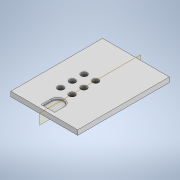
# Autodesk Inventor part: Part2
Saved by Autodesk Inventor 2022.6 (Build 266554010, 554A)
## iProperties
Created: 2025-05-13
Part Number: Part2
Material: Generic
Document SubType Name: Modeling
Designer: khinm
Density: 1 g/cm^3
Appearance: Default
Author: khinm
Autodesk Inventor part; units mm, degrees
ref_plane "XZ Plane" through (0, 0, 0) normal (0, 1, 0) x (-1, 0, 0)
ref_plane "XY Plane" through (0, 0, 0) normal (0, 0, 1) x (1, 0, 0)
sketch "Sketch1" plane through (0, 0, 0) normal (0, 0, 1) x (1, 0, 0)
  line L0 (-37.75, 2.75) -> (37.75, 2.75)
  line L1 (37.75, 2.75) -> (37.75, -2.75)
  line L2 (37.75, -2.75) -> (-37.75, -2.75)
  line L3 (-37.75, -2.75) -> (-37.75, 2.75)
  point P0 (0, 0)
  point P1 (0, 2.75)
  point P2 (-37.75, 0)
  dimension "d0" = 5.5
  dimension "d1" = 75.5
  constraints: 8 end point, 2 midpoint, 2 parallel, 1 horizontal, 1 horizontal alignment, 1 perpendicular, 1 vertical alignment
  measures "d0" distance of L0.end L1.end
  measures "d1" distance of L0.start L0.end
extrude "Extrusion1" add sketch "Sketch1" along normal mid plane 103.5
ref_plane "Work Plane1" through (0, 0, 0) normal (1, 0, 0) x (0, 1, 0)
sketch "Sketch6" plane through (0, 0, 0) normal (1, 0, 0) x (0, 1, 0)
  line L0 (-2.75, 51.75) -> (-2.75, -51.75) projected
  line L1 (-2.75, 49.5) -> (-4.75, 48.3453)
  line L2 (-4.75, 48.3453) -> (-4.75, 47.6547)
  line L3 (-4.75, 47.6547) -> (-2.75, 46.5)
  line L4 (-2.75, 46.5) -> (-2.75, 49.5)
  point P0 (0, 0)
  point P1 (-2.75, 48)
  point P2 (-4.75, 48)
  dimension "d17" = 2.25
  dimension "d18" = 3
  dimension "d19" = 2
  dimension "d20" = 60
  constraints: 8 end point, 2 midpoint, 2 parallel, 1 horizontal alignment, 1 point on line
  measures "d17" distance of L1.start L0.start
  measures "d18" distance of L3.end L1.start
  measures "d19" distance of point (-2.75, 48) point (-4.75, 48)
  measures "d20" angle of L0 L1
extrude "Extrusion4" add sketch "Sketch6" along normal mid plane 59.9
sketch "Sketch7" plane through (-37.75, 2.75, 51.75) normal (0, 1, 0) x (1, 0, 0)
  line L0 (75.5, 0) -> (0, 0) projected
  line L1 (44.3814, 15) -> (44.3814, 5)
  line L2 (44.3814, 5) -> (31.1186, 5)
  line L3 (31.1186, 5) -> (31.1186, 15)
  arc A0 (44.3814, 15) -> (31.1186, 15) centre (37.75, 15) ccw
  point P0 (37.75, 51.75)
  point P1 (37.75, 5)
  point P2 (37.75, 0)
  point P3 (37.75, 0)
  dimension "d23" = 5
  dimension "d25" = 10
  dimension "d26" = 6.6314
  constraints: 6 end point, 3 midpoint, 2 parallel, 2 point on circle, 2 vertical alignment, 1 centre point, 1 horizontal alignment
  measures "d23" distance between parallel lines of L2 L0
  measures "d25" distance of L1.end L1.start
  measures "d26" radius of A0
extrude "Extrusion5" cut sketch "Sketch7" against normal blind 2
chamfer "Chamfer2" distance 1 angle 45 4 edges at (0, 2.75, 30.1186) (6.6314, 2.75, 41.75) (-6.6314, 2.75, 41.75) (0, 2.75, 46.75)
sketch "Sketch8" plane through (-37.75, 2.75, 51.75) normal (0, 1, 0) x (1, 0, 0)
  line L0 (0, 103.5) -> (75.5, 103.5) projected
  line L1 (3, 100.5) -> (72.5, 100.5)
  line L2 (72.5, 100.5) -> (72.5, 6)
  line L3 (72.5, 6) -> (3, 6)
  line L4 (3, 6) -> (3, 100.5)
  line L5 (0, 103.5) -> (0, 0) projected
  line L6 (75.5, 0) -> (0, 0) projected
  line L7 (9.25, 96.25) -> (66.25, 96.25)
  line L8 (66.25, 96.25) -> (66.25, 10.25)
  line L9 (66.25, 10.25) -> (9.25, 10.25)
  line L10 (9.25, 10.25) -> (9.25, 96.25)
  line L11 (18.25, 71.25) -> (44.25, 71.25)
  line L12 (44.25, 71.25) -> (44.25, 18.25)
  line L13 (44.25, 18.25) -> (18.25, 18.25)
  line L14 (18.25, 18.25) -> (18.25, 71.25)
  line L15 (18.25, 44.75) -> (44.25, 44.75)
  line L16 (18.25, 58) -> (44.25, 58)
  line L17 (18.25, 31.5) -> (44.25, 31.5)
  circle A0 centre (24.75, 58) radius 3
  circle A1 centre (24.75, 44.75) radius 3
  circle A2 centre (24.75, 31.5) radius 3
  circle A3 centre (37.75, 58) radius 3
  circle A4 centre (37.75, 44.75) radius 3
  circle A5 centre (37.75, 31.5) radius 3
  point P0 (37.75, 51.75)
  point P1 (37.75, 100.5)
  point P2 (37.75, 103.5)
  point P3 (37.75, 96.25)
  point P4 (3, 53.25)
  point P5 (9.25, 53.25)
  point P6 (31.25, 31.5)
  dimension "d32" = 3
  dimension "d33" = 3
  dimension "d34" = 6
  dimension "d35" = 57
  dimension "d36" = 86
  dimension "d37" = 8
  dimension "d38" = 53
  dimension "d39" = 26
  dimension "d40" = 22
  dimension "d44" = 6.5
  dimension "d45" = 6.5
  dimension "d46" = 6.5
  dimension "d47" = 6.5
  dimension "d48" = 6.5
  dimension "d49" = 6.5
  dimension "d50" = 6
  dimension "d51" = 6
  dimension "d52" = 6
  dimension "d53" = 6
  dimension "d54" = 6
  dimension "d55" = 6
  dimension "d56" = 13.25
  dimension "d57" = 26.5
  dimension "d58" = 13.25
  constraints: 30 end point, 10 point on line, 8 midpoint, 6 centre point, 6 coincident, 6 parallel, 5 perpendicular, 3 horizontal, 2 vertical alignment, 1 horizontal alignment
  measures "d32" distance between parallel lines of L0 L1
  measures "d33" distance between parallel lines of L5 L4
  measures "d34" distance between parallel lines of L3 L6
  measures "d35" distance of L7.start L7.end
  measures "d36" distance of L7.end L8.end
  measures "d37" distance between parallel lines of L13 L9
  measures "d38" distance of L11.end L12.end
  measures "d39" distance of L12.end L13.end
  measures "d40" distance between parallel lines of L8 L12
  measures "d44" distance of L16.start point (24.75, 58)
  measures "d45" distance of L16.end point (37.75, 58)
  measures "d46" distance of L15.start point (24.75, 44.75)
  measures "d47" distance of L15.end point (37.75, 44.75)
  measures "d48" distance of L17.start point (24.75, 31.5)
  measures "d49" distance of L17.end point (37.75, 31.5)
  measures "d50" diameter of A0
  measures "d51" diameter of A1
  measures "d52" diameter of A2
  measures "d53" diameter of A3
  measures "d54" diameter of A4
  measures "d55" diameter of A5
  measures "d56" distance from line of L11 A0.centre
  measures "d57" distance of L15.start L11.start
  measures "d58" distance from line of L13 point (31.25, 31.5)
extrude "Extrusion6" cut sketch "Sketch8" against normal up to surface (5.5 mm away) contours A0 L16 | L16 A0 | A3 L16 | L16 A3 | A1 L15 | L15 A1 | A4 L15 | L15 A4 | A2 L17 | L17 A2 | A5 L17 | L17 A5
chamfer "Chamfer3" distance 0.5 angle 45 6 edges at (-16, 2.75, -6.25) (-16, 2.75, 7) (-16, 2.75, 20.25) (-3, 2.75, 20.25) (-3, 2.75, 7) (-3, 2.75, -6.25)
body "Solid1"
